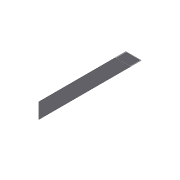
# Autodesk Inventor part: Frame_VerticalFrontAngle
Saved by Autodesk Inventor 2012 (Build 160160000, 160)
## iProperties
Created: 2012-01-21
Part Number: Frame_VerticalFrontAngle
Material: Aluminum-6061
Document SubType Name: Modeling
Designer: JesseK
Mass: 546.839 g
Surface Area: 336.02 cm^2
Volume: 201.786 cm^3
Density: 2.71 g/cm^3
Author: JesseK
Autodesk Inventor part; units mm, degrees
ref_plane "YZ Plane" through (0, 0, 0) normal (1, 0, 0) x (0, 1, 0)
ref_plane "XZ Plane" through (0, 0, 0) normal (0, 1, 0) x (-1, 0, 0)
ref_plane "XY Plane" through (0, 0, 0) normal (0, 0, 1) x (1, 0, 0)
sketch "Sketch1" plane through (0, 0, 0) normal (0, 0, 1) x (1, 0, 0)
  line L0 (0, 0) -> (0, 35.921)
  line L1 (0, 35.921) -> (177.8, 213.721)
  line L2 (177.8, 213.721) -> (213.721, 213.721)
  line L3 (213.721, 213.721) -> (0, 0)
  dimension "d0" = 25.4
  dimension "d2" = 177.8
  dimension "d3" = 177.8
  constraints: 8 end point, 1 horizontal, 1 parallel, 1 vertical
  measures "d0" distance between parallel lines of L3 L1
  measures "d2" distance from line of L2 L0.end
  measures "d3" horizontal distance of L1.end L0.end
extrude "Extrusion1" add sketch "Sketch1" along normal blind 25.4
shell "Shell1" thickness 1.5875 removed faces 2 at (0, 11.9737, 8.4667) at (189.7737, 213.721, 16.9333)
body "Solid1"
